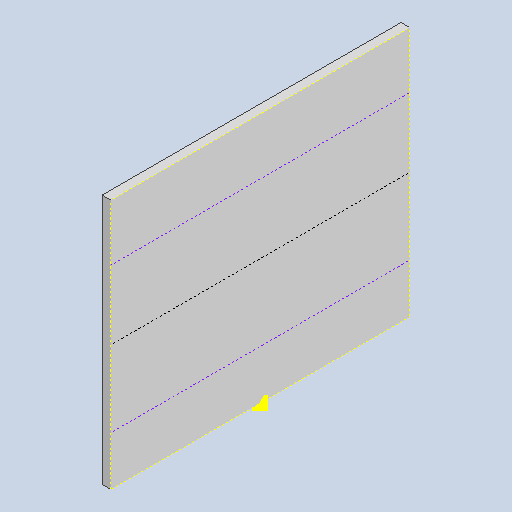
# Autodesk Inventor part: back_cowl
Saved by Autodesk Inventor 2025.2 (Build 292293000, 293)
## iProperties
Created: 2025-07-11
Part Number: back_cowl
Material: 일반
Document SubType Name: Modeling
Designer: jbhma
Density: 1 g/cm^3
Appearance: 기본값
Author: jbhma
Autodesk Inventor part; units mm, degrees
ref_plane "YZ Plane" through (0, 0, 0) normal (1, 0, 0) x (0, 1, 0)
ref_plane "XZ Plane" through (0, 0, 0) normal (0, 1, 0) x (-1, 0, 0)
ref_plane "XY Plane" through (0, 0, 0) normal (0, 0, 1) x (1, 0, 0)
sketch "스케치1" plane through (0, 0, 0) normal (1, 0, 0) x (0, 1, 0)
  line L0 (285, 170) -> (0, 170)
  line L1 (0, 170) -> (0, -170)
  line L2 (0, -170) -> (285, -170)
  line L3 (285, -170) -> (285, 170)
  point P0 (0, 0)
  point P1 (0, 0)
  dimension "d0" = 285
  dimension "d1" = 340
  constraints: 8 end point, 2 parallel, 1 coincident, 1 horizontal, 1 midpoint, 1 perpendicular
  measures "d0" distance between parallel lines of L3 L1
  measures "d1" distance of L0.end L1.end
extrude "돌출1" add sketch "스케치1" along normal blind 10
sketch "스케치2" plane through (10, 0, 0) normal (1, 0, 0) x (0, 0, -1)
  line L0 (-170, 0) -> (170, 0) construction
  line L1 (170, 0) -> (170, 285) construction
  line L2 (170, 285) -> (-170, 285) construction
  line L3 (-170, 285) -> (-170, 0) construction
  line L4 (-170, 142.5) -> (170, 142.5) construction
  line L5 (-170, 221) -> (170, 221) construction
  line L6 (-170, 56) -> (170, 56) construction
  point P0 (0, 0)
  constraints: 6 end point, 4 point on line, 2 midpoint, 2 perpendicular
